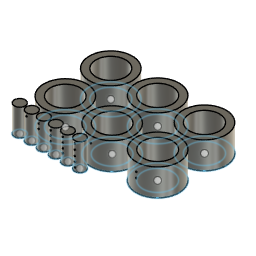
bearing test pieces (Autodesk Fusion 360 design; units mm, degrees)
Autodesk Fusion 360 part; units mm, degrees
sketch "Sketch1" plane through (0, 0, 0) normal (0, 0, 1) x (1, 0, 0)
  circle A0 centre (5.1375, 4.8167) radius 4
  circle A1 centre (14.1375, 4.8167) radius 3.975
  circle A2 centre (23.1375, 4.8167) radius 3.95
  circle A3 centre (32.1375, 4.8167) radius 3.925
  circle A4 centre (41.1375, 4.8167) radius 3.9
  circle A5 centre (50.1375, 4.8167) radius 3.875
  circle A6 centre (17.846, 26.1312) radius 11
  circle A7 centre (17.846, 26.1312) radius 16
  circle A8 centre (52.846, 26.1312) radius 16
  circle A9 centre (52.846, 26.1312) radius 11.025
  circle A10 centre (86.846, 26.1312) radius 11.05
  circle A11 centre (86.846, 26.1312) radius 16
  circle A12 centre (16.846, 61.1312) radius 11.075
  circle A13 centre (16.846, 61.1312) radius 16
  circle A14 centre (51.846, 61.1312) radius 11.1
  circle A15 centre (51.846, 61.1312) radius 16
  circle A16 centre (86.846, 61.1312) radius 11.125
  circle A17 centre (86.846, 61.1312) radius 16
  dimension "d1" = 8
  dimension "d2" = 7.95
  dimension "d3" = 7.9
  dimension "d4" = 7.85
  dimension "d5" = 7.8
  dimension "d6" = 7.75
  dimension "d8" = 22
  dimension "d9" = 32
  dimension "d10" = 22.05
  dimension "d11" = 32
  dimension "d12" = 22.1
  dimension "d13" = 32
  dimension "d14" = 22.15
  dimension "d15" = 32
  dimension "d16" = 22.2
  dimension "d17" = 32
  dimension "d18" = 22.25
  dimension "d19" = 32
  constraint concentric A6 A7
  constraint concentric A8 A9
  constraint concentric A10 A11
  constraint concentric A12 A13
  constraint concentric A14 A15
  constraint concentric A16 A17
  measures "d1" diameter of A0
  measures "d2" diameter of A1
  measures "d3" diameter of A2
  measures "d4" diameter of A3
  measures "d5" diameter of A4
  measures "d6" diameter of A5
  measures "d8" diameter of A6
  measures "d9" diameter of A7
  measures "d10" diameter of A9
  measures "d11" diameter of A8
  measures "d12" diameter of A10
  measures "d13" diameter of A11
  measures "d14" diameter of A12
  measures "d15" diameter of A13
  measures "d16" diameter of A14
  measures "d17" diameter of A15
  measures "d18" diameter of A16
  measures "d19" diameter of A17
extrude "Extrude1" add sketch "Sketch1" along normal blind 20 makes body 1 at (102.8261, 60.3337, 13.3333) makes body 2 at (9.1325, 4.6173, 13.3333) makes body 3 at (45.0326, 4.6223, 13.3333) makes body 4 at (36.0576, 4.621, 13.3333) makes body 5 at (33.8261, 25.3337, 13.3333) makes body 6 at (68.8261, 25.3337, 13.3333) makes body 7 at (67.8261, 60.3337, 13.3333) makes body 8 at (18.1075, 4.6185, 13.3333) makes body 9 at (54.0077, 4.6235, 13.3333) makes body 10 at (27.0826, 4.6198, 13.3333) makes body 11 at (32.8261, 60.3337, 13.3333) makes body 12 at (102.8261, 25.3337, 13.3333)
hole "Hole1" at (14.1375, 0.8417, 17.7895) direction (0, 1, 0) diameter 1 depth 1 tip angle 118 bodies 8
hole "Hole2" at (23.1375, 0.8667, 17.6874) direction (0, 1, 0) diameter 1 depth 1 tip angle 118 bodies 10
hole "Hole3" at (23.1375, 0.8667, 14.1905) direction (0, 1, 0) diameter 1 depth 1 tip angle 118 bodies 10
hole "Hole4" at (32.1375, 0.8917, 17.7217) direction (0, 1, 0) diameter 1 depth 1 tip angle 118 bodies 4
hole "Hole5" at (32.1375, 0.8917, 14.1805) direction (0, 1, 0) diameter 1 depth 1 tip angle 118 bodies 4
hole "Hole6" at (32.1375, 0.8917, 10.5447) direction (0, 1, 0) diameter 1 depth 1 tip angle 118 bodies 4
hole "Hole7" at (41.1375, 0.9167, 17.9542) direction (0, 1, 0) diameter 1 depth 1 tip angle 118 bodies 3
hole "Hole8" at (41.1375, 0.9167, 14.2574) direction (0, 1, 0) diameter 1 depth 1 tip angle 118 bodies 3
hole "Hole9" at (41.1375, 0.9167, 10.5198) direction (0, 1, 0) diameter 1 depth 1 tip angle 118 bodies 3
hole "Hole10" at (41.1375, 0.9167, 7.321) direction (0, 1, 0) diameter 1 depth 1 tip angle 118 bodies 3
hole "Hole11" at (50.1375, 0.9417, 18.1412) direction (0, 1, 0) diameter 1 depth 1 tip angle 118 bodies 9
hole "Hole12" at (50.1375, 0.9417, 14.1189) direction (0, 1, 0) diameter 1 depth 1 tip angle 118 bodies 9
hole "Hole13" at (50.1375, 0.9417, 10.0077) direction (0, 1, 0) diameter 1 depth 1 tip angle 118 bodies 9
hole "Hole14" at (50.1375, 0.9417, 6.3826) direction (0, 1, 0) diameter 1 depth 1 tip angle 118 bodies 9
hole "Hole15" at (50.1375, 0.9417, 2.7132) direction (0, 1, 0) diameter 1 depth 1 tip angle 118 bodies 9
hole "Hole16" at (52.846, 10.1312, 15.2126) direction (0, 1, 0) diameter 1 depth 1 tip angle 118 bodies 6
hole "Hole17" at (86.846, 10.1312, 13.6172) direction (0, 1, 0) diameter 1 depth 1 tip angle 118 bodies 12
hole "Hole18" at (86.846, 10.1312, 9.5333) direction (0, 1, 0) diameter 1 depth 1 tip angle 118 bodies 12
hole "Hole19" at (16.846, 77.1312, 14.5814) direction (0, -1, 0) diameter 1 depth 1 tip angle 118 bodies 11
hole "Hole20" at (16.846, 77.1312, 11.3047) direction (0, -1, 0) diameter 1 depth 1 tip angle 118 bodies 11
hole "Hole21" at (16.846, 77.1312, 7.7432) direction (0, -1, 0) diameter 1 depth 1 tip angle 118 bodies 11
hole "Hole22" at (51.846, 77.1312, 16.7183) direction (0, -1, 0) diameter 1 depth 1 tip angle 118 bodies 7
hole "Hole23" at (51.846, 77.1312, 13.0143) direction (0, -1, 0) diameter 1 depth 1 tip angle 118 bodies 7
hole "Hole24" at (51.846, 77.1312, 9.5952) direction (0, -1, 0) diameter 1 depth 1 tip angle 118 bodies 7
hole "Hole25" at (51.846, 77.1312, 6.0811) direction (0, -1, 0) diameter 1 depth 1 tip angle 118 bodies 7
hole "Hole26" at (86.846, 77.1312, 17.4666) direction (0, -1, 0) diameter 1 depth 1 tip angle 118 bodies 1
hole "Hole27" at (86.846, 77.1312, 13.5242) direction (0, -1, 0) diameter 1 depth 1 tip angle 118 bodies 1
hole "Hole28" at (86.846, 77.1312, 9.7443) direction (0, -1, 0) diameter 1 depth 1 tip angle 118 bodies 1
hole "Hole29" at (86.846, 77.1312, 6.0863) direction (0, -1, 0) diameter 1 depth 1 tip angle 118 bodies 1
hole "Hole30" at (86.846, 77.1312, 2.5909) direction (0, -1, 0) diameter 1 depth 1 tip angle 118 bodies 1
